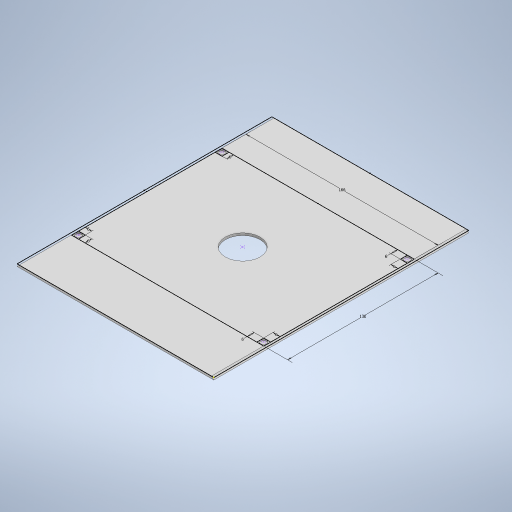
# Autodesk Inventor part: lid
Saved by Autodesk Inventor 2024 (Build 280153020, 153B)
## iProperties
Created: 2025-07-14
Part Number: lid
Material: Generic
Document SubType Name: Modeling
Designer: andre
Density: 1 g/cm^3
Appearance: Default
Author: andre
Autodesk Inventor part; units mm, degrees
ref_plane "YZ Plane" through (0, 0, 0) normal (1, 0, 0) x (0, 1, 0)
ref_plane "XZ Plane" through (0, 0, 0) normal (0, 1, 0) x (-1, 0, 0)
ref_plane "XY Plane" through (0, 0, 0) normal (0, 0, 1) x (1, 0, 0)
sketch "Sketch1" plane through (0, 0, 0) normal (0, 1, 0) x (-1, 0, 0)
  line L0 (0, 0) -> (170, 0)
  line L1 (170, 0) -> (170, -220)
  line L2 (170, -220) -> (0, -220)
  line L3 (0, -220) -> (0, 0)
  dimension "d0" = 170
  dimension "d1" = 220
  constraints: 8 end point, 2 parallel, 1 horizontal, 1 perpendicular
  measures "d0" distance of L1.end L2.end
  measures "d1" distance of L0.end L1.end
extrude "base" add sketch "Sketch1" along normal blind 2
chamfer "chamfers" distance 2 angle 45 2 edges at (-170, 2, -110) (0, 2, -110)
sketch "holes" plane through (0, 2, 0) normal (0, 1, 0) x (1, 0, 0)
  line L0 (-170, 220) -> (-170, 0) projected
  line L1 (0, 220) -> (-170, 220) projected
  line L2 (-170, 0) -> (0, 0)
  line L3 (0, 0) -> (0, 220)
  line L4 (0, 220) -> (-170, 220)
  line L5 (-170, 220) -> (-170, 0)
  line L6 (-168, 45) -> (-2, 45)
  line L7 (-2, 45) -> (-2, 175)
  line L8 (-2, 175) -> (-168, 175)
  line L9 (-168, 175) -> (-168, 45)
  line L10 (-2, 45) -> (-8, 45)
  line L11 (-8, 45) -> (-8, 51)
  line L12 (-8, 51) -> (-2, 51)
  line L13 (-2, 51) -> (-2, 45)
  line L14 (-2, 175) -> (-8, 175)
  line L15 (-8, 175) -> (-8, 169)
  line L16 (-8, 169) -> (-2, 169)
  line L17 (-2, 169) -> (-2, 175)
  line L18 (-168, 45) -> (-162, 45)
  line L19 (-162, 45) -> (-162, 51)
  line L20 (-162, 51) -> (-168, 51)
  line L21 (-168, 51) -> (-168, 45)
  line L22 (-168, 175) -> (-162, 175)
  line L23 (-162, 175) -> (-162, 169)
  line L24 (-162, 169) -> (-168, 169)
  line L25 (-168, 169) -> (-168, 175)
  point P0 (-85, 175)
  point P1 (-85, 220)
  point P2 (-168, 110)
  point P3 (-170, 110)
  point P4 (-165, 48)
  point P5 (-165, 172)
  point P6 (-5, 172)
  point P7 (-5, 48)
  point P8 (-85, 110)
  dimension "d10" = 166
  dimension "d11" = 130
  dimension "d12" = 6
  dimension "d13" = 6
  dimension "d14" = 6
  dimension "d15" = 6
  dimension "d16" = 6
  dimension "d17" = 6
  dimension "d18" = 6
  constraints: 48 end point, 12 parallel, 6 horizontal, 6 perpendicular, 4 midpoint, 1 horizontal alignment, 1 point on line, 1 vertical alignment
  measures "d10" distance of L8.end L7.end
  measures "d11" distance of L7.end L6.end
  measures "d12" distance of L11.end L12.end
  measures "d13" distance of L10.end L11.end
  measures "d14" distance of L16.end L15.end
  measures "d15" distance of L15.end L14.end
  measures "d16" distance of L20.end L19.end
  measures "d17" distance of L19.end L18.end
  measures "d18" distance of L22.end L23.end
hole "magnet_holders" at (-165, 2, -48) at (-165, 2, -172) at (-5, 2, -172) at (-5, 2, -48) direction (0, -1, 0) diameter 5.5 depth 1
hole "wire_hole" at (-85, 2, -110) direction (0, -1, 0) diameter 30 end through all
body "Solid1"
